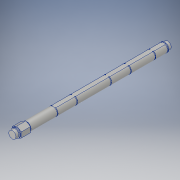
# Autodesk Inventor part: Column Axle
Saved by Autodesk Inventor 2019.4 (Build 234330000, 330)
## iProperties
Created: 2020-01-23
Part Number: Column Axle
Material: Aluminum 6061
Document SubType Name: Modeling
Designer: admin
Density: 2.7 g/cm^3
Appearance: Aluminum - Flat
Mass: 53.1021 g
Surface Area: 120.089 cm^2
Volume: 19.6675 cm^3
Author: admin
Autodesk Inventor part; units mm, degrees
ref_plane "YZ Plane" through (0, 0, 0) normal (1, 0, 0) x (0, 1, 0)
ref_plane "XZ Plane" through (0, 0, 0) normal (0, 1, 0) x (-1, 0, 0)
ref_plane "XY Plane" through (0, 0, 0) normal (0, 0, 1) x (1, 0, 0)
sketch "Sketch1" plane through (0, 0, 0) normal (1, 0, 0) x (0, 1, 0)
  line L0 (0, 0) -> (5, 0)
  line L1 (5, 0) -> (5, -4)
  line L2 (5, -4) -> (6.15, -4)
  line L3 (5.9, -4.9) -> (5.9, -6)
  line L4 (5.9, -6) -> (7.5, -6)
  line L5 (7.5, -6) -> (7.5, -18.649)
  line L6 (6, -55.9) -> (5.65, -55.9)
  line L7 (5.65, -55.9) -> (5.65, -57)
  line L8 (5.65, -57) -> (6, -57)
  line L9 (6, -57) -> (6, -83)
  line L10 (6, -83) -> (5.65, -83)
  line L11 (5.65, -83) -> (5.65, -84.1)
  line L12 (5.65, -84.1) -> (6, -84.1)
  line L13 (6, -84.1) -> (6, -129.9)
  line L14 (6, -129.9) -> (5.65, -129.9)
  line L15 (5.65, -129.9) -> (5.65, -131)
  line L16 (5.65, -131) -> (6, -131)
  line L17 (6, -131) -> (6, -157)
  line L18 (6, -157) -> (5.65, -157)
  line L19 (5.65, -157) -> (5.65, -158.1)
  line L20 (5.65, -158.1) -> (6, -158.1)
  line L21 (6, -158.1) -> (6, -190.9)
  line L22 (6, -190.9) -> (5.65, -190.9)
  line L23 (5.65, -190.9) -> (5.65, -192)
  line L24 (5.65, -192) -> (6, -192)
  line L25 (6, -192) -> (6, -208)
  line L26 (6, -208) -> (5.65, -208)
  line L27 (5.65, -208) -> (5.65, -209.1)
  line L28 (5.65, -209.1) -> (6, -209.1)
  line L29 (6, -209.1) -> (6, -210)
  line L30 (6, -210) -> (5, -210)
  line L31 (5, -210) -> (5, -214)
  line L32 (5, -214) -> (0, -214)
  line L33 (0, -214) -> (0, 0)
  line L34 (5.9, -4.9) -> (6.15, -4.9)
  line L35 (6.15, -4.9) -> (6.15, -4)
  line L36 (6, -55.9) -> (6, -19.749)
  line L37 (6, -19.749) -> (5.65, -19.749)
  line L38 (5.65, -19.749) -> (5.65, -18.649)
  line L39 (5.65, -18.649) -> (7.5, -18.649)
  dimension "d0" = 5
  dimension "d1" = 7.5
  dimension "d2" = 1.6
  dimension "d4" = 0.35
  dimension "d5" = 1.1
  dimension "d6" = 1.1
  dimension "d7" = 1.1
  dimension "d8" = 1.1
  dimension "d9" = 1.1
  dimension "d10" = 1.1
  dimension "d11" = 4
  dimension "d12" = 1.1
  dimension "d13" = 2
  dimension "d14" = 5
  dimension "d15" = 12.649
  dimension "d16" = 4
  dimension "d19" = 6
  dimension "d20" = 26
  dimension "d21" = 16
  dimension "d23" = 26
  dimension "d24" = 57
  dimension "d26" = 2
  dimension "d35" = 57
  dimension "d36" = 206
  dimension "d44" = 5.9
  dimension "d45" = 0.25
  dimension "d46" = 1.1
  constraints: 80 end point, 23 perpendicular, 20 point on line, 2 collinear, 2 horizontal, 2 vertical
  measures "d0" distance of L0.start L0.end
  measures "d1" distance between parallel lines of L33 L5
  measures "d2" distance of L3.end L4.end
  measures "d4" distance of L6.start L6.end
  measures "d5" distance of L6.end L7.end
  measures "d6" distance of L10.end L11.end
  measures "d7" distance of L14.end L15.end
  measures "d8" distance of L18.end L19.end
  measures "d9" distance of L22.end L23.end
  measures "d10" distance of L26.end L27.end
  measures "d11" distance of L0.end L1.end
  measures "d12" distance of L3.start L3.end
  measures "d13" distance between parallel lines of L2 L4
  measures "d14" distance between parallel lines of L33 L31
  measures "d15" distance of L4.end L5.end
  measures "d16" distance of L30.end L31.end
  measures "d19" distance between parallel lines of L33 L9
  measures "d20" distance of L8.end L9.end
  measures "d21" distance of L24.end L25.end
  measures "d23" distance of L16.end L17.end
  measures "d24" distance between parallel lines of L0 L8
  measures "d26" distance between parallel lines of L30 L26
  measures "d35" distance between parallel lines of L32 L18
  measures "d36" distance between parallel lines of L30 L2
  measures "d44" distance between parallel lines of L33 L3
  measures "d45" distance of L3.start L34.end
  measures "d46" distance of L37.end L38.end
revolve "Revolution1" add sketch "Sketch1" angle 360 about axis through (0, 0, -214) along (0, 0, 1)
sketch "Sketch3" plane through (0, 0, -18.649) normal (0, 0, -1) x (-1, 0, 0)
  line L0 (0, 7.3323) -> (6.35, 3.6662)
  line L1 (6.35, 3.6662) -> (6.35, -3.6662)
  line L2 (6.35, -3.6662) -> (0, -7.3323)
  line L3 (0, -7.3323) -> (-6.35, -3.6662)
  line L4 (-6.35, -3.6662) -> (-6.35, 3.6662)
  line L5 (-6.35, 3.6662) -> (0, 7.3323)
  circle A0 centre (0, 0) radius 7.5 projected
  point P0 (0, 0)
  point P1 (0, 0)
  dimension "d37" = 12.7
  constraints: 12 end point, 1 coincident, 13 other
  measures "d37" distance between parallel lines of L1 L4
extrude "Extrusion1" cut sketch "Sketch3" against normal up to surface (12.649 mm away)
sketch "Sketch4" plane through (0, 0, -55.9) normal (0, 0, 1) x (1, 0, 0)
  circle A0 centre (0, 0) radius 5.65 construction
  circle A1 centre (0, 0) radius 6 projected
  line L0 (-2.9047, 5.25) -> (2.9047, 5.25)
  point P0 (0, 0)
  dimension "d42" = 5.25
  constraints: 2 end point, 2 point on circle, 1 horizontal
  measures "d42" distance from line of A0.centre L0
extrude "Extrusion2" cut sketch "Sketch4" against normal up to surface (153.2 mm away) contours L0 A1 picked at (-0.2018, 5.4898)
body "Solid1"
